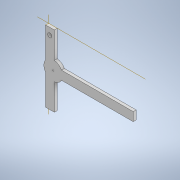
# Autodesk Inventor part: P3
Saved by Autodesk Inventor 2022 (Build 260153000, 153)
## iProperties
Created: 2022-11-21
Part Number: P3
Material: Genérico
Document SubType Name: Modeling
Designer: javie
Density: 1 g/cm^3
Appearance: Valor por defecto
Author: javie
Autodesk Inventor part; units mm, degrees
ref_plane "YZ Plane" through (0, 0, 0) normal (1, 0, 0) x (0, 1, 0)
ref_plane "XZ Plane" through (0, 0, 0) normal (0, 1, 0) x (-1, 0, 0)
ref_plane "XY Plane" through (0, 0, 0) normal (0, 0, 1) x (1, 0, 0)
sketch "Boceto1" plane through (0, 0, 0) normal (0, 0, 1) x (1, 0, 0)
  line L0 (0, -51.6726) -> (0, 0)
  line L1 (0, 0) -> (15, 0)
  line L2 (15, 0) -> (15, -45.1255)
  circle A0 centre (7.2527, -11.7) radius 3.5
  arc A1 (0, -51.6726) -> (0, -70.3274) centre (13, -61) ccw
  line L3 (27.1333, -53.5) -> (150, -53.5)
  line L4 (150, -53.5) -> (150, -68.5)
  line L5 (150, -68.5) -> (27.1333, -68.5)
  line L6 (15, -76.8745) -> (15, -122)
  line L7 (15, -122) -> (0, -122)
  line L8 (0, -122) -> (0, -70.3274)
  arc A2 (15, -76.8745) -> (27.1333, -68.5) centre (13, -61) ccw
  arc A3 (27.1333, -53.5) -> (15, -45.1255) centre (13, -61) ccw
  circle A4 centre (13, -61) radius 1
  point P0 (0, -70.3274)
  point P1 (15, -76.8745)
  dimension "d0" = 2
  constraints: 18 end point, 6 point on circle, 5 centre point, 1 coincident
  measures "d0" diameter of A4
extrude "Extrusión1" add sketch "Boceto1" along normal blind 5
